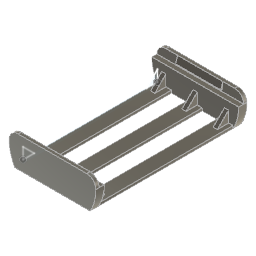
board_seat_SCC (Autodesk Fusion 360 design; units mm, degrees)
Autodesk Fusion 360 part; units mm, degrees
note: some values were not read from the file. Chosen so that the rebuilt part matches the saved one: which bodies a step acts on.
sketch "Sketch1" plane through (0, 0, 0) normal (0, 1, 0) x (1, 0, 0)
  circle A0 centre (0, -75) radius 31.25
  line L0 (0, -75) -> (-31.25, -75)
  line L1 (31.25, -75) -> (0, -75)
  line L2 (0, -43.75) -> (0, -59.375) construction
  line L3 (0, -59.375) -> (27.0633, -59.375)
  line L4 (0, -59.375) -> (-27.0633, -59.375)
  dimension "d1" = 62.5
  dimension "d3" = 15.625
  constraint coincident A0.centre L0.start
  constraint coincident A0 L0.end
  constraint horizontal L0
  constraint coincident A0 L1.start
  constraint parallel L0 L1
  constraint coincident A0 L2.start
  constraint perpendicular L1 L2
  constraint coincident A0 L3.end
  constraint perpendicular L2 L3
  constraint coincident A0 L4.end
  constraint perpendicular L2 L4
  measures "d1" diameter of A0
  measures "d3" distance of L2.start L2.end
extrude "Extrude1" add sketch "Sketch1" along normal blind 108.6 contours A0 L0 L1 L3 L4 makes body 1
extrude "Extrude2" cut 1 faces at (-9.0211, 0, 64.5833) along direction (0, 1, 0) blind 96.6 from surface at 6 on bodies 1 bodies 1 makes body 2 at (9.0211, 102.6, 69.7917)
sketch "Sketch2" plane through (0, 0, 0) normal (0, -1, 0) x (1, 0, 0)
  arc A0 (27.0633, 59.375) -> (31.25, 75) centre (0, 75) ccw
  line L0 (31.25, 75) -> (-31.25, 75)
  arc A1 (-31.25, 75) -> (-27.0633, 59.375) centre (0, 75) ccw
  line L1 (-27.0633, 59.375) -> (27.0633, 59.375)
  line L2 (-27.0633, 59.375) -> (-17.0633, 59.375)
  line L3 (-17.0633, 59.375) -> (-17.0633, 60.875)
  line L4 (-17.0633, 60.875) -> (-27.0633, 60.875)
  line L5 (-27.0633, 60.875) -> (-27.0633, 59.375)
  line L6 (27.0633, 59.375) -> (17.0633, 59.375)
  line L7 (17.0633, 59.375) -> (17.0633, 60.875)
  line L8 (17.0633, 60.875) -> (27.0633, 60.875)
  line L9 (27.0633, 60.875) -> (27.0633, 59.375)
  line L10 (0, 59.375) -> (-5, 59.375) construction
  line L11 (-5, 59.375) -> (-5, 60.875) construction
  line L12 (-5, 60.875) -> (0, 60.875) construction
  line L13 (0, 60.875) -> (0, 59.375) construction
  line L14 (-5, 60.875) -> (5, 60.875)
  line L15 (5, 60.875) -> (5, 59.375)
  line L16 (5, 59.375) -> (-5, 59.375)
  line L17 (-5, 59.375) -> (-5, 60.875)
  dimension "d9" = 10
  dimension "d10" = 1.5
  dimension "d11" = 10
  dimension "d12" = 1.5
  dimension "d13" = 5
  dimension "d14" = 1.5
  dimension "d15" = 10
  constraint horizontal L2
  constraint vertical L3
  constraint horizontal L4
  constraint vertical L5
  constraint coincident A1.end L1.start
  constraint horizontal L6
  constraint vertical L7
  constraint horizontal L8
  constraint vertical L9
  constraint coincident A0.start L1.end
  constraint horizontal L10
  constraint vertical L11
  constraint horizontal L12
  constraint vertical L13
  constraint midpoint L1 L10.start
  constraint horizontal L14
  constraint vertical L15
  constraint horizontal L16
  constraint vertical L17
  measures "d9" distance of A1.end L2.end
  measures "d10" distance of A1.end L4.end
  measures "d11" distance of A0.start L6.end
  measures "d12" distance of A0.start L8.end
  measures "d13" distance of L10.start L10.end
  measures "d14" distance of L10.start L12.end
  measures "d15" distance of L11.end L14.end
extrude "Extrude3" add sketch "Sketch2" against normal blind 105 contours L1 L6 L7 L8 L9 | L1 L14 L15 L16 L17 | L1 L2 L3 L4 L5 bodies 1 2
sketch "Sketch3" plane through (0, 0, 75) normal (0, 0, 1) x (-1, 0, 0)
  line L0 (31.25, -102.6) -> (-31.25, -102.6)
  line L1 (-31.25, -102.6) -> (-31.25, -108.6)
  line L2 (-31.25, -108.6) -> (31.25, -108.6)
  line L3 (31.25, -108.6) -> (31.25, -102.6)
  line L4 (31.25, -108.6) -> (-31.25, -108.6)
  line L5 (-31.25, -108.6) -> (-31.25, -106.2)
  line L6 (-31.25, -106.2) -> (31.25, -106.2)
  line L7 (31.25, -106.2) -> (31.25, -108.6)
  line L8 (31.25, 0) -> (-31.25, 0) construction
  line L9 (-31.25, 0) -> (-31.25, -6) construction
  line L10 (-31.25, -6) -> (31.25, -6) construction
  line L11 (31.25, -6) -> (31.25, 0) construction
  line L12 (31.25, 0) -> (-31.25, 0)
  line L13 (-31.25, 0) -> (-31.25, -2.4)
  line L14 (-31.25, -2.4) -> (31.25, -2.4)
  line L15 (31.25, -2.4) -> (31.25, 0)
  dimension "d18" = 2.4
  dimension "d19" = 2.4
  constraint horizontal L4
  constraint vertical L5
  constraint horizontal L6
  constraint vertical L7
  constraint coincident L2.end L3.start
  constraint horizontal L8
  constraint vertical L9
  constraint horizontal L10
  constraint vertical L11
  constraint horizontal L12
  constraint vertical L13
  constraint horizontal L14
  constraint vertical L15
  measures "d18" distance of L2.end L6.end
  measures "d19" distance of L8.start L14.end
extrude "Extrude4" add sketch "Sketch3" along normal blind 6.6 contours L1 L2 L3 L4 L5 L6 L7 | L12 L13 L14 L15 bodies 1
sketch "Sketch4" plane through (-31.25, 0, 0) normal (-1, 0, 0) x (0, -1, 0)
  line L0 (-108.6, 75) -> (-106.2, 75)
  line L1 (-106.2, 75) -> (-106.2, 81.6)
  line L2 (-106.2, 81.6) -> (-108.6, 81.6)
  line L3 (-108.6, 81.6) -> (-108.6, 75)
  line L4 (-106.2, 81.6) -> (-106.2, 77)
  line L5 (-106.2, 77) -> (-104.7, 77)
  line L6 (-104.7, 77) -> (-106.2, 81.6)
  line L7 (-2.4, 75) -> (-2.4, 81.6)
  line L8 (-2.4, 81.6) -> (-2.4, 77)
  line L9 (-2.4, 77) -> (-3.9, 77)
  line L10 (-3.9, 77) -> (-2.4, 81.6)
  dimension "d22" = 4.6
  dimension "d23" = 1.5
  dimension "d24" = 4.6
  dimension "d25" = 1.5
  constraint coincident L1.end L2.start
  constraint perpendicular L0 L4
  constraint perpendicular L4 L5
  constraint coincident L7.end L8.start
  constraint parallel L7 L8
  constraint perpendicular L8 L9
  measures "d22" distance of L1.end L4.end
  measures "d23" distance of L4.end L5.end
  measures "d24" distance of L7.end L8.end
  measures "d25" distance of L8.end L9.end
extrude "Extrude5" add sketch "Sketch4" against normal blind 32.5 from surface at -15 contours L1 L4 L5 L6 | L7 L8 L9 L10 bodies 1
fillet "Fillet1" radius 6.6 4 edges at (-31.25, 1.2, 81.6) (-31.25, 107.4, 81.6) (31.25, 107.4, 81.6) (31.25, 1.2, 81.6) on bodies 1
extrude "Extrude6" add 3 faces at (-20.3966, 38.2, 60.875) (-1.6667, 38.2, 60.875) (20.3966, 38.2, 60.875) along direction (0, 0, 1) blind 0.5 on bodies 1 bodies 1
sketch "Sketch5" plane through (-27.0633, 0, 0) normal (-1, 0, 0) x (0, -1, 0)
  line L0 (-102.6, 61.375) -> (-102.6, 59.375)
  line L1 (-102.6, 59.375) -> (-6, 59.375)
  line L2 (-6, 59.375) -> (-6, 61.375)
  line L3 (-6, 61.375) -> (-102.6, 61.375)
  line L4 (-102.6, 61.375) -> (-102.6, 69.375)
  line L5 (-102.6, 61.375) -> (-94.6, 61.375)
  line L6 (-94.6, 61.375) -> (-102.6, 69.375)
  line L7 (-6, 61.375) -> (-6, 69.375)
  line L8 (-6, 61.375) -> (-14, 61.375)
  line L9 (-14, 61.375) -> (-6, 69.375)
  dimension "d33" = 8
  dimension "d34" = 8
  dimension "d35" = 8
  dimension "d36" = 8
  constraint coincident L0.start L3.end
  constraint perpendicular L3 L4
  constraint perpendicular L4 L5
  constraint coincident L2.end L3.start
  constraint perpendicular L3 L7
  constraint perpendicular L7 L8
  measures "d33" distance of L0.start L4.end
  measures "d34" distance of L0.start L5.end
  measures "d35" distance of L2.end L7.end
  measures "d36" distance of L2.end L8.end
extrude "Extrude7" add sketch "Sketch5" against normal blind 3 from surface at -3 contours L3 L4 L5 L6 | L3 L7 L8 L9 bodies 1
extrude "Extrude8" add sketch "Sketch5" against normal blind 3 from surface at -48 contours L3 L4 L5 L6 | L3 L7 L8 L9 bodies 1
extrude "Extrude9" add sketch "Sketch5" against normal blind 3 from surface at -25.5 contours L3 L4 L5 L6 | L3 L7 L8 L9 bodies 1
